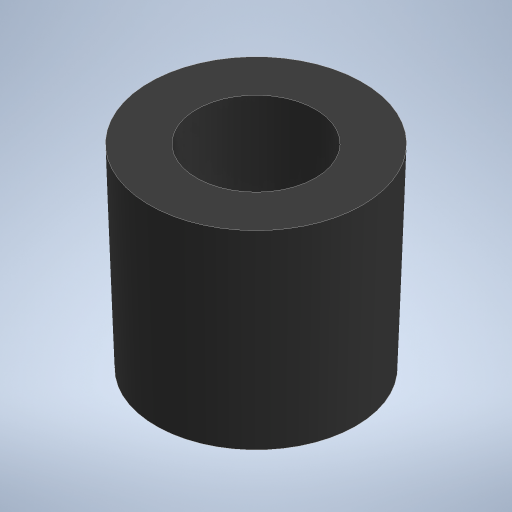
# Autodesk Inventor part: Pata-Goma
Saved by Autodesk Inventor 2023.1 (Build 271208000, 208)
## iProperties
Created: 2023-05-02
Part Number: Pata-Goma
Material: Rubber
Document SubType Name: Modeling
Designer: felip
Density: 0.93 g/cm^3
Appearance: Rubber - Black
Author: felip
Autodesk Inventor part; units mm, degrees
ref_plane "YZ Plane" through (0, 0, 0) normal (1, 0, 0) x (0, 1, 0)
ref_plane "XZ Plane" through (0, 0, 0) normal (0, 1, 0) x (-1, 0, 0)
ref_plane "XY Plane" through (0, 0, 0) normal (0, 0, 1) x (1, 0, 0)
sketch "Sketch1" plane through (0, 0, 0) normal (0, 0, 1) x (1, 0, 0)
  line L0 (0, 0) -> (9.25, 0)
  line L1 (9.25, 0) -> (9.85, 18)
  line L2 (9.85, 18) -> (0, 18)
  line L3 (0, 18) -> (0, 0)
  dimension "d0" = 9.85
  dimension "d1" = 9.25
  dimension "d2" = 18
  constraints: 8 end point, 1 horizontal, 1 parallel, 1 perpendicular
  measures "d0" distance of L1.end L2.end
  measures "d1" distance of L0.start L0.end
  measures "d2" distance of L2.end L0.start
revolve "Revolution1" add sketch "Sketch1" angle 360 about axis through (0, 18, 0) along (0, -1, 0)
sketch "Sketch2" plane through (0, 18, 0) normal (0, 1, 0) x (1, 0, 0)
  circle A0 centre (0, 0) radius 4.64
  dimension "d4" = 9.28
  constraints: 1 centre point, 1 coincident
  measures "d4" diameter of A0
hole "Hole1" at (0, 18, 0) direction (0, -1, 0) diameter 11 end through all
body "Solid1"
